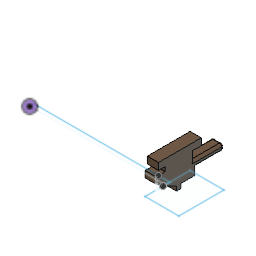
T Shape Projectile (Autodesk Fusion 360 design; units mm, degrees)
part number: 2026-05-27-21-05-35-437
Autodesk Fusion 360 part; units mm, degrees
sketch "Sketch9" plane through (0, 0, 0) normal (0, 1, 0) x (1, 0, 0)
  line L0 (0, 0) -> (60, 0)
  line L1 (0, 0) -> (0, 2)
  line L2 (0, 2) -> (60, 2)
  line L3 (60, 2) -> (60, 0)
  line L4 (60, 1) -> (60, 11)
  line L5 (60, 1) -> (60, -9)
  line L6 (60, 11) -> (75, 11)
  line L7 (75, 11) -> (75, -9)
  line L8 (75, -9) -> (60, -9)
  dimension "d108" = 60
  dimension "d109" = 10
  constraint coincident L0.start L1.start
  constraint horizontal L0
  constraint perpendicular L0 L1
  constraint perpendicular L1 L2
  constraint midpoint L3 L4.start
  constraint perpendicular L2 L4
  constraint perpendicular L0 L5
  constraint perpendicular L4 L6
  constraint perpendicular L6 L7
  measures "d108" distance of L0.start L0.end
  measures "d109" distance of L4.start L5.end
extrude "Extrude38" add sketch "Sketch9" along normal blind 2 contours L0 L1 L2 L3 L4 L5
extrude "Extrude39" add sketch "Sketch9" along normal blind 20 contours L3 L4 L5 L6 L7 L8
sketch "Sketch10" plane through (75, 0, 0) normal (1, 0, 0) x (0, 0, -1)
  line L0 (-9, 0) -> (11, 0)
  line L1 (11, 0) -> (11, 20)
  line L2 (11, 20) -> (-9, 20)
  line L3 (-9, 20) -> (-9, 0)
  line L4 (-9, 0) -> (-6, 0)
  line L5 (-6, 0) -> (-6, 3)
  line L6 (-6, 3) -> (-9, 3)
  line L7 (-9, 0) -> (-9, 3)
  line L8 (11, 0) -> (11, 3)
  line L9 (11, 3) -> (8, 3)
  line L10 (8, 3) -> (8, 0)
  line L11 (11, 0) -> (8, 0)
  constraint coincident L0.start L3.end
  constraint coincident L0 L4.end
  constraint perpendicular L4 L5
  constraint coincident L3 L6.end
  constraint perpendicular L3 L6
  constraint coincident L0.end L1.start
  constraint coincident L1 L8.end
  constraint perpendicular L8 L9
  constraint coincident L0 L10.end
  constraint perpendicular L0 L10
extrude "Extrude40" cut sketch "Sketch10" against normal blind 19 contours L0 L3 L4 L5 L6 L7 | L0 L1 L8 L9 L10 L11
sketch "Sketch11" plane through (60, 0, 0) normal (-1, 0, 0) x (0, 0, 1)
  line L0 (6, 0) -> (6, 3)
  line L1 (6, 3) -> (9, 3)
  line L2 (9, 3) -> (9, 20)
  line L3 (9, 20) -> (-11, 20)
  line L4 (-11, 20) -> (-11, 3)
  line L5 (-11, 3) -> (-8, 3)
  line L6 (-8, 3) -> (-8, 0)
  line L7 (-8, 0) -> (-2, 0)
  line L8 (-2, 0) -> (-2, 2)
  line L9 (-2, 2) -> (0, 2)
  line L10 (0, 2) -> (0, 0)
  line L11 (0, 0) -> (6, 0)
  line L12 (6, 0) -> (6, 2)
  line L13 (6, 2) -> (0, 2)
  line L14 (0, 0) -> (6, 0)
  line L15 (6, 0) -> (6, 2)
  line L16 (6, 2) -> (0, 2)
  line L17 (0, 2) -> (0, 0)
  line L18 (-2, 2) -> (-8, 2)
  line L19 (-8, 2) -> (-8, 0)
  line L20 (-8, 0) -> (-2, 0)
  line L21 (-2, 0) -> (-2, 2)
  constraint coincident L0.start L11.end
  constraint coincident L0 L12.end
  constraint coincident L9.end L10.start
  constraint horizontal L14
  constraint vertical L15
  constraint horizontal L16
  constraint vertical L17
  constraint coincident L10.end L11.start
  constraint horizontal L18
  constraint vertical L19
  constraint horizontal L20
  constraint vertical L21
  constraint coincident L6.end L7.start
  constraint coincident L8.end L9.start
extrude "Extrude41" cut sketch "Sketch11" against normal blind 59 contours L0 L10 L11 L12 L13 L14 L15 L16 L17 | L6 L7 L8 L18 L19 L20 L21
sketch "Sketch12" plane through (60, 0, 0) normal (-1, 0, 0) x (0, 0, 1)
  line L0 (-8, 2) -> (-2, 2)
  line L1 (-2, 2) -> (0, 2)
  line L2 (0, 2) -> (6, 2)
  line L3 (6, 2) -> (6, 3)
  line L4 (6, 3) -> (9, 3)
  line L5 (9, 3) -> (9, 20)
  line L6 (9, 20) -> (-11, 20)
  line L7 (-11, 20) -> (-11, 3)
  line L8 (-11, 3) -> (-8, 3)
  line L9 (-8, 3) -> (-8, 2)
  line L10 (-11, 3) -> (-8, 3)
  line L11 (-8, 3) -> (-8, 6)
  line L12 (-8, 6) -> (-11, 6)
  line L13 (-11, 6) -> (-11, 3)
  line L14 (9, 3) -> (6, 3)
  line L15 (6, 3) -> (6, 6)
  line L16 (6, 6) -> (9, 6)
  line L17 (9, 6) -> (9, 3)
  dimension "d118" = 3
  dimension "d119" = 3
  dimension "d120" = 3
  dimension "d121" = 3
  constraint horizontal L10
  constraint vertical L11
  constraint horizontal L12
  constraint vertical L13
  constraint coincident L7.end L8.start
  constraint horizontal L14
  constraint vertical L15
  constraint horizontal L16
  constraint vertical L17
  constraint coincident L4.end L5.start
  measures "d118" distance of L7.end L8.end
  measures "d119" distance of L7.end L12.end
  measures "d120" distance of L4.end L3.end
  measures "d121" distance of L4.end L16.end
extrude "Extrude42" cut sketch "Sketch12" against normal blind 28 contours L7 L8 L10 L11 L12 L13 | L4 L5 L14 L15 L16 L17
extrude "Extrude43" add 2 faces at (65, 6, 7) (65, 6, -9) along direction (0, -1, 0) blind 1
extrude "Extrude44" cut 1 faces at (0, 0.6667, -0.6667) along direction (1, 0, 0) blind 55
extrude "Extrude45" cut 1 faces at (75, 15, 1.3333) along direction (-1, 0, 0) blind 5
extrude "Extrude46" cut 1 faces at (66.6667, 20, -0.6667) along direction (0, -1, 0) blind 5
sketch "Sketch13" plane through (0, 0, -11) normal (0, 0, -1) x (-1, 0, 0)
  line L0 (-60, 15) -> (-70, 15)
  line L1 (-70, 15) -> (-70, 5)
  line L2 (-70, 5) -> (-60, 5)
  line L3 (-60, 5) -> (-60, 15)
  line L4 (-60, 15) -> (-60, 12)
  line L5 (-60, 12) -> (-70, 12)
  line L6 (-70, 12) -> (-70, 8)
  line L7 (-70, 8) -> (-60, 8)
  line L8 (-60, 8) -> (-60, 12)
  constraint coincident L0.start L3.end
  constraint coincident L3 L4.end
  constraint horizontal L5
  constraint vertical L6
  constraint horizontal L7
  constraint vertical L8
  constraint coincident L1 L6.end
sketch "Sketch14" plane through (0, 0, 9) normal (0, 0, 1) x (1, 0, 0)
  line L0 (70, 15) -> (60, 15)
  line L1 (60, 15) -> (60, 5)
  line L2 (60, 5) -> (70, 5)
  line L3 (70, 5) -> (70, 15)
  line L4 (70, 12) -> (60, 12)
  line L5 (60, 12) -> (60, 8)
  line L6 (60, 8) -> (70, 8)
  line L7 (70, 8) -> (70, 12)
  constraint horizontal L4
  constraint vertical L5
  constraint horizontal L6
  constraint vertical L7
  constraint coincident L1 L5.end
  constraint coincident L3 L4.start
extrude "Extrude47" cut sketch "Sketch14" against normal blind 4 contours L1 L3 L4 L5 L6 L7
extrude "Extrude48" cut sketch "Sketch13" against normal blind 4 contours L1 L3 L5 L6 L7 L8
extrude "Extrude49" add 1 faces at (66.6667, 6, -11) along direction (0, 0, -1) blind 10
extrude "Extrude50" cut 1 faces at (70, 6, -1.3333) along direction (-1, 0, 0) blind 5
fillet "Fillet12" radius 1 4 edges at (60, 6.5, -21) (65, 6.5, -21) (62.5, 8, -21) (62.5, 5, -21)
fillet "Fillet13" radius 1 4 edges at (60, 8, -13.5) (60.2929, 7.7071, -20.7071) (60, 5, -14) (60.2929, 5.2929, -20.7071)
fillet "Fillet14" radius 1 4 edges at (65, 8, -13.5) (64.7071, 7.7071, -20.7071) (64.7071, 5.2929, -20.7071) (65, 5, -14)
extrude "Extrude51" cut 1 faces at (55, 0.6667, -0.6667) along direction (1, 0, 0) blind 3
extrude "Extrude52" add 1 faces at (61.6667, 8, 7.6667) along direction (0, 1, 0) blind 2
extrude "Extrude53" cut 2 faces at (61.6667, 8.6667, 9) (61.6667, 6, 9) along direction (0, 0, -1) blind 1
extrude "Extrude54" cut 1 faces at (61.6667, 14, 9) along direction (0, 0, -1) blind 1
sketch "Sketch17" plane through (65, 0, 0) normal (1, 0, 0) x (0, 0, -1)
  line L0 (-8, 15) -> (-8, 12)
  line L1 (-8, 12) -> (-5, 12)
  line L2 (-5, 12) -> (-5, 10)
  line L3 (-5, 10) -> (-8, 10)
  line L4 (-8, 10) -> (-8, 5)
  line L5 (-8, 5) -> (-6, 5)
  line L6 (-6, 5) -> (-6, 2)
  line L7 (-6, 2) -> (0, 2)
  line L8 (0, 2) -> (0, 0)
  line L9 (0, 0) -> (2, 0)
  line L10 (2, 0) -> (2, 2)
  line L11 (2, 2) -> (8, 2)
  line L12 (8, 2) -> (8, 6)
  line L13 (8, 6) -> (20, 6)
  line L14 (20, 6) -> (20, 7)
  line L15 (20, 7) -> (7, 7)
  line L16 (7, 7) -> (7, 12)
  line L17 (7, 12) -> (11, 12)
  line L18 (11, 12) -> (11, 15)
  line L19 (11, 15) -> (-8, 15)
  line L20 (0, 2) -> (-6.002, 5)
  line L21 (-6.002, 5) -> (-6, 2)
  line L22 (0, 2) -> (-6, 2)
  dimension "d199" = 6.71
  constraint coincident L7.end L8.start
  constraint coincident L5 L20.end
  constraint coincident L6.end L7.start
  measures "d199" distance of L7.end L20.end
extrude "Extrude57" cut sketch "Sketch17" against normal blind 8.5 contours L6 L7 L20 L21 L22
sketch "Sketch18" plane through (65, 0, 0) normal (1, 0, 0) x (0, 0, -1)
  line L0 (-6, 4.999) -> (0, 2)
  line L1 (0, 2) -> (0, 0)
  line L2 (0, 0) -> (2, 0)
  line L3 (2, 0) -> (2, 2)
  line L4 (2, 2) -> (8, 2)
  line L5 (8, 2) -> (8, 6)
  line L6 (8, 6) -> (20, 6)
  line L7 (20, 6) -> (20, 7)
  line L8 (20, 7) -> (7, 7)
  line L9 (7, 7) -> (7, 12)
  line L10 (7, 12) -> (11, 12)
  line L11 (11, 12) -> (11, 15)
  line L12 (11, 15) -> (-8, 15)
  line L13 (-8, 15) -> (-8, 12)
  line L14 (-8, 12) -> (-5, 12)
  line L15 (-5, 12) -> (-5, 10)
  line L16 (-5, 10) -> (-8, 10)
  line L17 (-8, 10) -> (-8, 5)
  line L18 (-8, 5) -> (-6, 5)
  line L19 (-6, 5) -> (-6, 4.999)
  line L20 (-6, 5) -> (-9, 5)
  line L21 (-9, 5) -> (-9, 7.13)
  line L22 (-9, 7.13) -> (-6, 4.999)
  line L23 (-8, 10) -> (-9, 10)
  line L24 (-9, 10) -> (-9, 7.13)
  dimension "d202" = 3
  dimension "d203" = 2.13
  constraint coincident L18.end L19.start
  constraint perpendicular L17 L20
  constraint perpendicular L20 L21
  constraint coincident L0.start L19.end
  constraint coincident L16.end L17.start
  constraint perpendicular L17 L23
  constraint perpendicular L16 L24
  measures "d202" distance of L18.end L20.end
  measures "d203" distance of L20.end L21.end
extrude "Extrude58" cut sketch "Sketch18" against normal blind 13 contours L17 L18 L20 L22
extrude "Extrude59" add sketch "Sketch18" against normal blind 5 contours L17 L22 L23 L24
